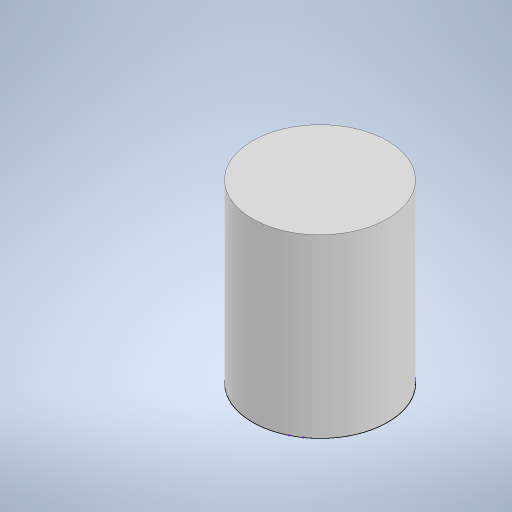
# Autodesk Inventor part: Medium Peg Part
Saved by Autodesk Inventor 2023.1 (Build 271208000, 208)
## iProperties
Created: 2022-09-22
Part Number: Medium Peg Part
Material: Generic
Document SubType Name: Modeling
Designer: petro
Density: 1 g/cm^3
Appearance: Default
Author: petro
Autodesk Inventor part; units mm, degrees
ref_plane "YZ Plane" through (0, 0, 0) normal (1, 0, 0) x (0, 1, 0)
ref_plane "XZ Plane" through (0, 0, 0) normal (0, 1, 0) x (-1, 0, 0)
ref_plane "XY Plane" through (0, 0, 0) normal (0, 0, 1) x (1, 0, 0)
sketch "Sketch1" plane through (0, 0, 0) normal (0, 1, 0) x (-1, 0, 0)
  circle A0 centre (0, 0) radius 1.15
  point P0 (1.1476, -0.075)
  point P1 (-0.5088, 1.0313)
  point P2 (-0.6588, 0.9426)
  point P3 (-0.7388, -0.8813)
  point P4 (-0.5088, -1.0313)
  point P5 (1.1476, 0.075)
  dimension "d41" = 2.3
  dimension "d46" = 0.15
  dimension "d57" = 0.15
  dimension "d59" = 0.15
  constraints: 6 point on circle, 1 centre point, 1 coincident
  measures "d41" diameter of A0
  measures "d46" distance of point (1.148, 0.075) point (1.148, -0.075)
  measures "d57" vertical distance of A0.end A0.start
  measures "d59" horizontal distance of point (-0.509, 1.031) point (-0.659, 0.943)
extrude "Extrusion3" add sketch "Sketch1" along normal blind 3
body "Solid2"
